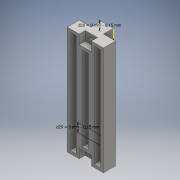
# Autodesk Inventor part: centerbeam
Saved by Autodesk Inventor 2016 (Build 200138000, 138)
## iProperties
Created: 2015-12-02
Part Number: centerbeam
Material: Generic
Document SubType Name: Modeling
Designer: hesaon
Density: 1 g/cm^3
Appearance: Default
Author: hesaon
Autodesk Inventor part; units mm, degrees
ref_plane "YZ Plane" through (0, 0, 0) normal (1, 0, 0) x (0, 1, 0)
ref_plane "XZ Plane" through (0, 0, 0) normal (0, 1, 0) x (-1, 0, 0)
ref_plane "XY Plane" through (0, 0, 0) normal (0, 0, 1) x (1, 0, 0)
sketch "Sketch1" plane through (0, 0, 0) normal (0, 0, 1) x (1, 0, 0)
  line L0 (0, 0) -> (36, 0)
  line L1 (36, 0) -> (36, 12)
  line L2 (36, 12) -> (24, 12)
  line L3 (24, 12) -> (24, 22)
  line L4 (24, 22) -> (12, 22)
  line L5 (12, 22) -> (12, 12)
  line L6 (12, 12) -> (0, 12)
  line L7 (0, 12) -> (0, 0)
  dimension "d0" = 36
  dimension "d1" = 12
  dimension "d2" = 12
  dimension "d3" = 10
  dimension "d4" = 12
  constraints: 16 end point, 6 perpendicular, 2 point on line, 1 horizontal
  measures "d0" distance of L0.start L0.end
  measures "d1" distance of L0.end L1.end
  measures "d2" distance of L1.end L2.end
  measures "d3" distance of L2.end L3.end
  measures "d4" distance of L3.end L4.end
extrude "Extrusion1" add sketch "Sketch1" along normal blind 108
sketch "Sketch2" plane through (0, 0, 0) normal (0, -1, 0) x (1, 0, 0)
  circle A0 centre (18, 4.5) radius 1.725
  line L0 (0, 0) -> (36, 0) projected
  line L1 (36, 0) -> (36, 108) projected
  circle A1 centre (18, 103.5) radius 1.725
  line L2 (0, 108) -> (36, 108) projected
  dimension "d7" = 3.45
  dimension "d8" = 4.5
  dimension "d9" = 18
  dimension "d10" = 3.45
  dimension "d11" = 18
  dimension "d12" = 4.5
  constraints: 2 centre point
  measures "d7" diameter of A0
  measures "d8" distance from line of L0 A0.centre
  measures "d9" distance from line of L1 A0.centre
  measures "d10" diameter of A1
  measures "d11" distance from line of L1 A1.centre
  measures "d12" distance from line of L2 A1.centre
extrude "Extrusion2" cut sketch "Sketch2" against normal blind 20
sketch "Sketch3" plane through (12, 22, 0) normal (0, 1, 0) x (1, 0, 0)
  circle A0 centre (6, -4.5) radius 1.725 projected
  circle A1 centre (6, -4.5) radius 3
  circle A2 centre (6, -103.5) radius 1.725 projected
  circle A3 centre (6, -103.5) radius 3
  point P0 (-12, 0)
  dimension "d15" = 6
  dimension "d16" = 6
  constraints: 2 centre point, 2 coincident
  measures "d15" diameter of A1
  measures "d16" diameter of A3
extrude "Extrusion3" cut sketch "Sketch3" against normal blind 2 contours A0 | A1 | A2 | A3
sketch "Sketch4" plane through (36, 0, 0) normal (1, 0, 0) x (0, 0, -1)
  line L0 (-108, 0) -> (-107.85, 0)
  line L1 (0, 0) -> (-108, 0) projected
  line L2 (-107.85, 0) -> (-107.85, 12)
  line L3 (0, 12) -> (-108, 12) projected
  line L4 (-108, 0) -> (-108, 12) projected
  line L5 (-108, 12) -> (-108, 0)
  line L6 (-108, 22) -> (-107.85, 22)
  line L7 (-107.85, 12) -> (-108, 12)
  line L8 (0, 0) -> (-0.15, 0)
  line L9 (-0.15, 0) -> (-0.15, 12)
  line L10 (-0.15, 12) -> (0, 12)
  line L11 (0, 12) -> (0, 0)
  line L12 (0, 22) -> (-0.15, 22)
  line L13 (-0.15, 12) -> (0, 12)
  dimension "d19" = 0.15
  dimension "d20" = 12
  dimension "d21" = 0.15
  dimension "d22" = 0.15
  constraints: 22 end point, 5 equal length, 3 horizontal, 3 point on line, 2 perpendicular
  measures "d19" distance of L0.start L0.end
  measures "d20" distance of L0.end L2.end
  measures "d21" distance of L3.end L2.end
  measures "d22" distance of L9.end L10.end
extrude "Extrusion4" cut sketch "Sketch4" against normal through all contours L4 L3 L2 L0 | L9 L3 L11 L1
sketch "Sketch5" plane through (24, 22, 108) normal (1, 0, 0) x (0, 0, -1)
  line L0 (108, -10) -> (108, 0) projected
  line L1 (108, 0) -> (0, 0) projected
  line L2 (108, -10) -> (107.85, -10)
  line L3 (107.85, -10) -> (107.85, 0)
  line L4 (107.85, 0) -> (108, 0)
  line L5 (108, 0) -> (108, -10)
  line L6 (0.15, -10) -> (0, -10) projected
  line L7 (0, -10) -> (0, 0) projected
  line L8 (0.15, -10) -> (0, -10)
  line L9 (0, -10) -> (0, 0)
  line L10 (0, 0) -> (0.15, 0)
  line L11 (0.15, 0) -> (0.15, -10)
  point P0 (108, -22)
  dimension "d25" = 0.15
  constraints: 16 end point, 4 parallel, 2 horizontal, 2 perpendicular, 1 point on line
  measures "d25" distance of L3.end L4.end
extrude "Extrusion5" cut sketch "Sketch5" against normal through all
sketch "Sketch6" plane through (12, 22, 0.15) normal (0, 1, 0) x (1, 0, 0)
  line L0 (0, 0) -> (0, -107.7) projected
  line L1 (12, 0) -> (12, -107.7) projected
  line L2 (0, -98.85) -> (12, -98.85)
  line L3 (12, -98.85) -> (12, -8.85)
  line L4 (12, -8.85) -> (0, -8.85)
  line L5 (0, -8.85) -> (0, -98.85)
  point P0 (-12, 0.15)
  dimension "d28" = 8.85
  dimension "d29" = 8.85
  constraints: 8 end point, 2 parallel, 2 point on line, 1 horizontal, 1 perpendicular
  measures "d28" distance of L0.end L2.start
  measures "d29" distance of L0.start L4.end
sketch "Sketch7" plane through (0, 0, 107.85) normal (0, -1, 0) x (1, 0, 0)
  line L0 (0, -107.7) -> (36, -107.7) projected
  line L1 (11.85, -107.7) -> (24.15, -107.7)
  line L2 (24.15, -107.7) -> (24.15, -98.55)
  line L3 (24.15, -98.55) -> (11.85, -98.55)
  line L4 (11.85, -98.55) -> (11.85, -107.7)
  line L5 (0, 0) -> (12, 0) projected
  line L6 (11.85, 0) -> (24.15, 0)
  line L7 (24.15, 0) -> (24.15, -9.15)
  line L8 (24.15, -9.15) -> (11.85, -9.15)
  line L9 (11.85, -9.15) -> (11.85, 0)
  line L10 (36, -107.7) -> (36, 0) projected
  point P0 (0, -107.85)
  dimension "d30" = 11.85
  dimension "d31" = 11.85
  dimension "d32" = 9.15
  dimension "d33" = 11.85
  dimension "d34" = 11.85
  dimension "d35" = 9.15
  constraints: 16 end point, 4 parallel, 2 horizontal, 2 perpendicular, 2 point on line
  measures "d30" distance of L1.start L0.start
  measures "d31" distance of L0.end L1.end
  measures "d32" distance of L2.end L1.end
  measures "d33" distance of L5.start L6.start
  measures "d34" distance from line of L10 L6.end
  measures "d35" distance of L6.end L7.end
extrude "Extrusion6" cut sketch "Sketch7" against normal blind 6
sketch "Sketch8" plane through (36, 0, 0.15) normal (0, -1, 0) x (1, 0, 0)
  line L0 (-21, 95.7) -> (-15, 95.7)
  line L1 (-15, 95.7) -> (-15, 12)
  line L2 (-15, 12) -> (-21, 12)
  line L3 (-21, 12) -> (-21, 95.7)
  line L4 (-11.85, 0) -> (-24.15, 0) projected
  line L5 (0, 107.7) -> (-11.85, 107.7) projected
  line L6 (-24, 0) -> (-24, 107.7) projected
  line L7 (-12, 0) -> (-12, 107.7) projected
  point P0 (-36, -0.15)
  dimension "d38" = 12
  dimension "d39" = 12
  dimension "d40" = 3
  dimension "d41" = 3
  constraints: 8 end point, 2 parallel, 1 horizontal, 1 perpendicular
  measures "d38" distance from line of L4 L1.end
  measures "d39" distance from line of L5 L0.end
  measures "d40" distance between parallel lines of L6 L3
  measures "d41" distance between parallel lines of L1 L7
extrude "Extrusion7" cut sketch "Sketch8" against normal through all
sketch "Sketch9" plane through (24, 12, 107.85) normal (0, 1, 0) x (1, 0, 0)
  line L0 (9, 3) -> (3, 3)
  line L1 (3, 3) -> (3, 104.7)
  line L2 (3, 104.7) -> (9, 104.7)
  line L3 (9, 104.7) -> (9, 3)
  line L4 (-15, 3) -> (-21, 3)
  line L5 (-21, 3) -> (-21, 104.7)
  line L6 (-21, 104.7) -> (-15, 104.7)
  line L7 (-15, 104.7) -> (-15, 3)
  line L8 (12, 0) -> (0.15, 0) projected
  line L9 (12, 107.7) -> (0, 107.7) projected
  line L10 (12, 107.7) -> (12, 0) projected
  line L11 (-24, 107.7) -> (-24, 0) projected
  line L12 (-12, 107.7) -> (-24, 107.7) projected
  line L13 (-24, 0) -> (-12, 0) projected
  line L14 (-12, 107.7) -> (-12, 0) projected
  line L15 (0, 107.7) -> (0, 0) projected
  point P0 (-24, 107.85)
  dimension "d44" = 3
  dimension "d45" = 3
  dimension "d46" = 3
  dimension "d47" = 3
  dimension "d48" = 3
  dimension "d49" = 3
  dimension "d50" = 3
  dimension "d51" = 3
  constraints: 16 end point, 4 parallel, 2 horizontal, 2 perpendicular
  measures "d44" distance between parallel lines of L8 L0
  measures "d45" distance between parallel lines of L9 L2
  measures "d46" distance between parallel lines of L3 L10
  measures "d47" distance between parallel lines of L11 L5
  measures "d48" distance between parallel lines of L12 L6
  measures "d49" distance between parallel lines of L13 L4
  measures "d50" distance between parallel lines of L14 L7
  measures "d51" distance between parallel lines of L15 L1
extrude "Extrusion8" cut sketch "Sketch9" against normal through all contours L0 L1 L2 L3 | L4 L5 L6 L7
body "Solid1"
